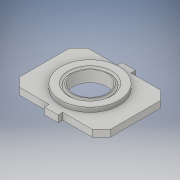
# Autodesk Inventor part: chamber_top
Saved by Autodesk Inventor 2019 (Build 230136000, 136)
## iProperties
Created: 2020-06-08
Part Number: chamber_top
Material: Generic
Document SubType Name: Modeling
Designer: honqi
Density: 1 g/cm^3
Appearance: Default
Author: honqi
Autodesk Inventor part; units mm, degrees
ref_plane "YZ Plane" through (0, 0, 0) normal (1, 0, 0) x (0, 1, 0)
ref_plane "XZ Plane" through (0, 0, 0) normal (0, 1, 0) x (-1, 0, 0)
ref_plane "XY Plane" through (0, 0, 0) normal (0, 0, 1) x (1, 0, 0)
sketch "Sketch1" plane through (0, 0, 0) normal (0, 1, 0) x (-1, 0, 0)
  line L0 (0, 0) -> (-40, 0)
  line L1 (-40, 0) -> (-40, -30)
  line L2 (-40, -30) -> (0, -30)
  line L3 (0, -30) -> (0, 0)
  dimension "d0" = 30
  dimension "d1" = 40
  constraints: 8 end point, 2 parallel, 1 horizontal, 1 perpendicular
  measures "d0" distance of L2.end L0.start
  measures "d1" distance of L1.end L2.end
extrude "Extrusion1" add sketch "Sketch1" along normal blind 3
sketch "Sketch2" plane through (0, 3, 0) normal (0, 1, 0) x (1, 0, 0)
  circle A0 centre (20, 15) radius 7.5
  line L0 (0, 30) -> (0, 0) projected
  line L1 (0, 0) -> (40, 0) projected
  dimension "d4" = 15
  dimension "d5" = 20
  dimension "d6" = 15
  constraints: 1 centre point
  measures "d4" diameter of A0
  measures "d5" distance from line of L0 A0.centre
  measures "d6" distance from line of L1 A0.centre
extrude "Extrusion2" cut sketch "Sketch2" against normal blind 3
sketch "Sketch3" plane through (0, 3, 0) normal (0, 1, 0) x (1, 0, 0)
  circle A0 centre (20, 15) radius 7.5 projected
  circle A1 centre (20, 15) radius 7.5
  circle A2 centre (20, 15) radius 12.8
  point P0 (0, 0)
  dimension "d9" = 25.6
  constraints: 2 centre point, 2 coincident
  measures "d9" diameter of A2
extrude "Extrusion3" add sketch "Sketch3" along normal blind 2
sketch "Sketch4" plane through (0, 0, 0) normal (0, -1, 0) x (1, 0, 0)
  circle A0 centre (5, -25) radius 2.368
  circle A1 centre (5, -5) radius 2.5
  circle A2 centre (35, -25) radius 2.5
  circle A3 centre (35, -5) radius 2.5
  circle A4 centre (20, -15) radius 7.5 projected
  point P0 (0, 0)
  dimension "d12" = 5
  dimension "d13" = 5
  dimension "d14" = 5
  dimension "d15" = 15
  dimension "d16" = 10
  dimension "d17" = 10
  dimension "d18" = 15
  dimension "d19" = 15
  dimension "d20" = 15
  dimension "d21" = 10
  dimension "d22" = 10
  constraints: 4 centre point, 1 coincident
  measures "d12" diameter of A1
  measures "d13" diameter of A2
  measures "d14" diameter of A3
  measures "d15" horizontal distance of A4.centre A0.centre
  measures "d16" vertical distance of A4.centre A0.centre
  measures "d17" vertical distance of point (20, -15) A1.centre
  measures "d18" horizontal distance of point (20, -15) A1.centre
  measures "d19" horizontal distance of point (20, -15) A2.centre
  measures "d20" horizontal distance of A4.centre A3.centre
  measures "d21" vertical distance of point (20, -15) A2.centre
  measures "d22" vertical distance of point (20, -15) A3.centre
extrude "Extrusion4" cut sketch "Sketch4" against normal blind 2 contours A0 | A1 | A2 | A3
chamfer "Chamfer1" distance 4 angle 45 4 edges at (40, 1.5, 0) (40, 1.5, -30) (0, 1.5, 0) (0, 1.5, -30)
sketch "Sketch5" plane through (0, 3, 0) normal (0, 1, 0) x (1, 0, 0)
  line L0 (36, 30) -> (4, 30) projected
  line L1 (17, 30) -> (23, 30)
  line L2 (23, 30) -> (23, 32)
  line L3 (23, 32) -> (17, 32)
  line L4 (17, 32) -> (17, 30)
  line L5 (17, 0) -> (23, 0)
  line L6 (23, 0) -> (23, -2)
  line L7 (23, -2) -> (17, -2)
  line L8 (17, -2) -> (17, 0)
  line L9 (0, 26) -> (0, 4) projected
  line L10 (4, 0) -> (36, 0) projected
  point P0 (0, 0)
  dimension "d28" = 6
  dimension "d29" = 17
  dimension "d30" = 2
  dimension "d31" = 6
  dimension "d32" = 17
  dimension "d33" = 2
  dimension "d34" = 0
  dimension "d35" = 2
  constraints: 16 end point, 4 parallel, 2 horizontal, 2 perpendicular, 1 point on line
  measures "d28" distance of L2.end L3.end
  measures "d29" distance between parallel lines of L9 L4
  measures "d30" distance of L1.end L2.end
  measures "d31" distance of L6.end L7.end
  measures "d32" distance between parallel lines of L9 L8
  measures "d33" distance of L5.end L6.end
  measures "d34" distance between parallel lines of L10 L5
  measures "d35" distance between parallel lines of L0 L3
extrude "Extrusion5" add sketch "Sketch5" against normal blind 3
sketch "Sketch6" plane through (20, 5, -15) normal (0, 1, 0) x (1, 0, 0)
  circle A0 centre (0, 0) radius 9.55
  circle A1 centre (0, 0) radius 7.9
  point P0 (-20, -15)
  dimension "d38" = 15.8
  dimension "d39" = 19.1
  constraints: 2 centre point, 1 coincident
  measures "d38" diameter of A1
  measures "d39" diameter of A0
extrude "Extrusion6" cut sketch "Sketch6" against normal blind 0.7
fillet "Fillet1" radius 0.8 2 edges at (12.1, 4.3, -15) (10.45, 4.3, -15)
body "Solid1"
